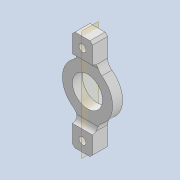
# Autodesk Inventor part: bearing_hh_1
Saved by Autodesk Inventor 2020 (Build 240168000, 168)
## iProperties
Created: 2021-09-09
Part Number: bearing_hh_1
Material: Generic
Document SubType Name: Modeling
Designer: Shuang Peng
Density: 1 g/cm^3
Appearance: Default
Author: Shuang Peng
Autodesk Inventor part; units mm, degrees
ref_plane "YZ Plane" through (0, 0, 0) normal (1, 0, 0) x (0, 1, 0)
ref_plane "XZ Plane" through (0, 0, 0) normal (0, 1, 0) x (-1, 0, 0)
ref_plane "XY Plane" through (0, 0, 0) normal (0, 0, 1) x (1, 0, 0)
sketch "Sketch1" plane through (0, 0, 0) normal (0, 0, 1) x (1, 0, 0)
  circle A0 centre (0, 0) radius 3 projected
  circle A1 centre (0, 0) radius 3
  circle A2 centre (0, 0) radius 5
  line L0 (0, 0) -> (0, 8)
  circle A3 centre (0, 8) radius 0.7
  line L1 (0, 0) -> (0, -8)
  circle A4 centre (0, -8) radius 0.7
  line L2 (-2, -10) -> (2, -10)
  line L3 (2, -10) -> (2, 10)
  line L4 (2, 10) -> (-2, 10)
  line L5 (-2, 10) -> (-2, -10)
  line L6 (-2, -10) -> (2, 10) construction
  line L7 (2, -10) -> (-2, 10) construction
  point P0 (-2, -4.5826)
  point P1 (2, -4.5826)
  point P2 (2, 4.5826)
  point P3 (-2, 4.5826)
  dimension "d0" = 6
  dimension "d1" = 10
  dimension "d2" = 8
  dimension "d3" = 1.4
  dimension "d4" = 8
  dimension "d5" = 1.4
  dimension "d6" = 4
  dimension "d7" = 20
  constraints: 16 end point, 4 centre point, 4 coincident, 2 midpoint, 2 parallel, 2 perpendicular, 2 vertical
  measures "d0" diameter of A1
  measures "d1" diameter of A2
  measures "d2" distance of L0.start L0.end
  measures "d3" diameter of A3
  measures "d4" distance of L0.start L1.end
  measures "d5" diameter of A4
  measures "d6" distance of L2.start L2.end
  measures "d7" distance of L3.end L2.end
extrude "Extrusion1" add sketch "Sketch1" against normal blind 2 contours A0 L3 A2 | A0 L0 A2 L3 | L3 A2 L1 A0 | A0 L5 A2 L0 | A2 L5 L4 L3 | L1 A2 L5 A0 | L3 L2 L5 A2 | A0 L5 A2
sketch "Sketch2" plane through (0, 0, 0) normal (0, 0, 1) x (1, 0, 0)
  arc A0 (-2, 4.5826) -> (-2, -4.5826) centre (0, 0) ccw projected
  line L0 (-2, -4.5826) -> (-2, -10) projected
  line L1 (-2, -10) -> (2, -10) projected
  line L2 (2, -10) -> (2, -4.5826) projected
  arc A1 (2, -4.5826) -> (2, 4.5826) centre (0, 0) ccw projected
  line L3 (2, 4.5826) -> (2, 10) projected
  line L4 (2, 10) -> (-2, 10) projected
  line L5 (-2, 10) -> (-2, 4.5826) projected
  circle A2 centre (0, -8) radius 0.7 projected
  circle A3 centre (0, 8) radius 0.7 projected
  circle A4 centre (0, 0) radius 3 projected
  line L6 (-2, -10) -> (-2, -4.5826) projected
  line L7 (-2, -10) -> (-2, -6)
  line L8 (-2, -6) -> (2, -6)
  line L9 (2, -10) -> (2, -4.5826) projected
  line L10 (-2, 10) -> (-2, 4.5826) projected
  line L11 (-2, 10) -> (-2, 6)
  line L12 (-2, 6) -> (2, 6)
  line L13 (2, 10) -> (2, 4.5826) projected
  point P0 (2, 6)
  dimension "d10" = 4
  dimension "d11" = 4
  constraints: 8 end point, 4 point on line, 1 horizontal, 1 perpendicular
  measures "d10" distance of L0.end L7.end
  measures "d11" distance of L4.end L11.end
extrude "Extrusion2" add sketch "Sketch2" along normal blind 1 contours L5 L4 L3 L12 | L8 L2 L1 L0
ref_plane "Work Plane1" through (0, -10, -2) normal (1, 0, 0) x (0, 0, -1)
chamfer "Chamfer1" distance 0.5 angle 45 4 edges at (-2, -10, -0.5) (2, -10, -0.5) (-2, 10, -0.5) (2, 10, -0.5)
fillet "Fillet1" radius 2 4 edges at (-2, -4.5826, -1) (-2, 4.5826, -1) (2, 4.5826, -1) (2, -4.5826, -1)
fillet "Fillet2" radius 1 2 edges at (0, -6, 0) (0, 6, 0)
body "Solid1"
